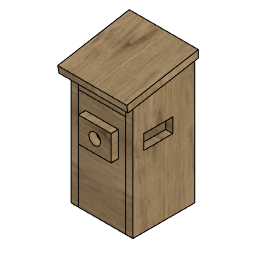
budka (Autodesk Fusion 360 design; units mm, degrees)
Autodesk Fusion 360 part; units mm, degrees
sketch "Szkic1" plane through (0, 0, 0) normal (0, 0, 1) x (1, 0, 0) in component "budka"
  line L0 (0, 0) -> (130, 0)
  line L1 (130, 0) -> (130, 130)
  line L2 (130, 130) -> (0, 130)
  line L3 (0, 130) -> (0, 0)
  constraint horizontal L0
  constraint vertical L1
  constraint horizontal L2
  constraint vertical L3
  constraint coincident L0.start L3.end
extrude "Wyciągnięcie proste1" add sketch "Szkic1" along normal blind 20 makes body 1 in component "budka"
sketch "Szkic2" plane through (0, 0, 0) normal (1, 0, 0) x (0, 1, 0) in component "budka"
  line L0 (-20, 0) -> (-20, 320)
  line L1 (-20, 320) -> (150, 350)
  line L2 (150, 350) -> (150, 0)
  line L3 (150, 0) -> (-20, 0)
  constraint vertical L0
  constraint parallel L0 L2
  constraint perpendicular L0 L3
extrude "Wyciągnięcie proste2" add sketch "Szkic2" against normal blind 20 separate body makes body 2 in component "budka"
copy_body "Kopiuj-wklej bryły1" bodies 2 makes body 3 in component "budka"
move_body "Przesuń1" bodies 3 to x (1, 0, 0) y (0, 1, 0) z (0, 0, 1) at (150, 0, 0) in component "budka"
sketch "Szkic4" plane through (0, 0, 0) normal (1, 0, 0) x (0, 1, 0) in component "budka"
  line L0 (130, 350) -> (130, 0)
  line L1 (130, 0) -> (150, 0)
  line L2 (150, 0) -> (150, 350)
  line L3 (150, 350) -> (130, 350)
  constraint vertical L0
  constraint perpendicular L0 L1
  constraint perpendicular L1 L2
  constraint perpendicular L0 L3
extrude "Wyciągnięcie proste3" add sketch "Szkic4" along normal blind 130 separate body makes body 4 in component "budka"
sketch "Szkic5" plane through (130, 0, 0) normal (1, 0, 0) x (0, 1, 0) in component "budka"
  line L0 (150, 350) -> (130, 350)
  line L1 (130, 350) -> (130, 0)
  line L2 (130, 0) -> (150, 0)
  line L3 (150, 0) -> (150, 350)
  line L4 (130, 350) -> (150, 350)
  line L5 (150, 350) -> (130, 346.4712)
  constraint coincident L0.end L1.start
  constraint coincident L0.start L3.end
  constraint coincident L1 L5.end
extrude "Wyciągnięcie proste4" cut sketch "Szkic5" against normal blind 132 contours L0 L1 L4 L5 bodies 4 in component "budka"
sketch "Szkic6" plane through (130, 0, 0) normal (-1, 0, 0) x (0, -1, 0) in component "budka"
  line L0 (-150, 350) -> (-150, 0)
  line L1 (-150, 0) -> (20, 0)
  line L2 (20, 0) -> (20, 320)
  line L3 (20, 320) -> (-150, 350)
  line L4 (20, 320) -> (0, 320)
  line L5 (0, 320) -> (0, 280)
  line L6 (0, 280) -> (20, 280)
  line L7 (20, 280) -> (20, 320)
  constraint horizontal L4
  constraint vertical L5
  constraint horizontal L6
  constraint vertical L7
  constraint coincident L2.end L3.start
extrude "Wyciągnięcie proste5" add sketch "Szkic6" along normal blind 130 separate body contours L2 L4 L5 L6 L7 makes body 5 in component "budka"
sketch "Szkic7" plane through (130, 0, 0) normal (-1, 0, 0) x (0, -1, 0) in component "budka"
  line L0 (-150, 350) -> (-150, 0)
  line L1 (-150, 0) -> (20, 0)
  line L2 (20, 0) -> (20, 320)
  line L3 (20, 320) -> (-150, 350)
  line L4 (0, 0) -> (20, 0)
  line L5 (20, 0) -> (20, 280)
  line L6 (20, 280) -> (0, 280)
  line L7 (0, 280) -> (0, 0)
  dimension "d11" = 280
  constraint horizontal L4
  constraint vertical L5
  constraint horizontal L6
  constraint vertical L7
  constraint coincident L2 L5.end
  constraint coincident L4.start L7.end
  measures "d11" distance of L1.end L5.end
extrude "Wyciągnięcie proste6" add sketch "Szkic7" along normal blind 130 separate body contours L1 L2 L4 L5 L6 L7 makes body 6 in component "budka"
copy_body "Kopiuj-wklej bryły2" bodies 1 makes body 7 in component "budka"
move_body "Przesuń2" bodies 7 to x (1, 0, 0) y (0, 1, 0) z (0, 0, 1) at (0, 0, 270) in component "budka"
sketch "Szkic8" plane through (0, -20, 0) normal (0, -1, 0) x (1, 0, 0) in component "budka"
  line L0 (130, 0) -> (130, 280)
  line L1 (130, 280) -> (0, 280)
  line L2 (0, 280) -> (0, 0)
  line L3 (0, 0) -> (130, 0)
  line L4 (20, 240) -> (110, 240)
  line L5 (110, 240) -> (110, 170)
  line L6 (110, 170) -> (20, 170)
  line L7 (20, 170) -> (20, 240)
  constraint horizontal L4
  constraint vertical L5
  constraint horizontal L6
  constraint vertical L7
extrude "Wyciągnięcie proste7" add sketch "Szkic8" along normal blind 20 separate body contours L4 L5 L6 L7 makes body 8 in component "budka"
copy_body "Kopiuj-wklej bryły3" bodies 8 makes body 9 in component "budka"
move_body "Przesuń3" bodies 9 to x (1, 0, 0) y (0, 1, 0) z (0, 0, 1) at (0, 40, 0) in component "budka"
sketch "Szkic9" plane through (0, -40, 0) normal (0, -1, 0) x (1, 0, 0) in component "budka"
  line L0 (20, 170) -> (110, 170)
  line L1 (110, 170) -> (110, 240)
  line L2 (110, 240) -> (20, 240)
  line L3 (20, 240) -> (20, 170)
  circle A0 centre (65, 205) radius 16
extrude "Wyciągnięcie proste8" cut sketch "Szkic9" against normal blind 76 contours A0 bodies 6 8 9 in component "budka"
sketch "Szkic10" plane through (150, 0, 0) normal (1, 0, 0) x (0, 1, 0) in component "budka"
  line L0 (150, 0) -> (150, 350)
  line L1 (150, 350) -> (-20, 320)
  line L2 (-20, 320) -> (-20, 0)
  line L3 (-20, 0) -> (150, 0)
  line L4 (10, 235) -> (90, 235)
  line L5 (90, 235) -> (90, 195)
  line L6 (90, 195) -> (10, 195)
  line L7 (10, 195) -> (10, 235)
  constraint horizontal L4
  constraint vertical L5
  constraint horizontal L6
  constraint vertical L7
extrude "Wyciągnięcie proste9" cut sketch "Szkic10" against normal blind 236 contours L4 L5 L6 L7 bodies 2 3 in component "budka"
ref_plane "Płaszczyzna konstrukcyjna1" through (65, 150, 350) normal (0, -0.173648, 0.984808) x (1, 0, 0) in component "budka"
sketch "Szkic11" plane through (0, -55.3305, 313.7947) normal (0, -0.173648, 0.984808) x (1, 0, 0) in component "budka"
  line L0 (-29.9995, 208) -> (160.0005, 208)
  line L1 (160.0005, 208) -> (160.0005, 8)
  line L2 (160.0005, 8) -> (-29.9995, 8)
  line L3 (-29.9995, 8) -> (-29.9995, 208)
  dimension "d21" = 190
  dimension "d22" = 200
  constraint horizontal L0
  constraint vertical L1
  constraint horizontal L2
  constraint vertical L3
  measures "d21" distance of L1.end L2.end
  measures "d22" distance of L0.end L1.end
extrude "Wyciągnięcie proste10" add sketch "Szkic11" along normal blind 20 separate body makes body 10 in component "budka"
move_body "Przesuń4" bodies 10 to x (1, 0, 0) y (0, 1, 0) z (0, 0, 1) at (0, 3.9392, 0.6946) in component "budka"
sketch "Szkic12" plane through (160.0005, 0, 0) normal (1, 0, 0) x (0, 1, 0) in component "budka"
  line L0 (-43.5128, 315.8785) -> (153.4488, 350.6081)
  line L1 (153.4488, 350.6081) -> (149.9758, 370.3043)
  line L2 (149.9758, 370.3043) -> (-46.9857, 335.5746)
  line L3 (-46.9857, 335.5746) -> (-43.5128, 315.8785)
  line L4 (149.9758, 370.3043) -> (149.9758, 349.9957)
  line L5 (153.4488, 350.6081) -> (149.9758, 370.3043)
  constraint coincident L1.end L2.start
  constraint coincident L0 L4.end
  constraint vertical L4
  constraint coincident L0.end L1.start
extrude "Wyciągnięcie proste11" cut sketch "Szkic12" against normal blind 207 contours L0 L1 L4 L5 bodies 10 in component "budka"
component "budka" placed x (1, 0, 0) y (0, 1, 0) z (0, 0, 1) at (-1.6546, -7.6761, -0.608)
named bodies: "podloga", "scianka lewo", "scianka prawo", "tyl", "ukryty sufit", "przedluzenie przod", "przedluzenie tyl", "dach"
